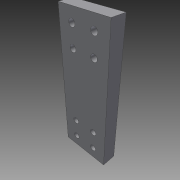
# Autodesk Inventor part: x_iddler_right_cap
Saved by Autodesk Inventor 2014 (Build 180170000, 170)
## iProperties
Created: 2014-03-25
Part Number: x_iddler_right_cap
Material: Plywood, Finish
Document SubType Name: Modeling
Designer: buben
Density: 0.552 g/cm^3
Appearance: Plywood - New
Author: buben
Autodesk Inventor part; units mm, degrees
ref_plane "YZ Plane" through (0, 0, 0) normal (1, 0, 0) x (0, 1, 0)
ref_plane "XZ Plane" through (0, 0, 0) normal (0, 1, 0) x (-1, 0, 0)
ref_plane "XY Plane" through (0, 0, 0) normal (0, 0, 1) x (1, 0, 0)
sketch "Sketch1" plane through (0, 0, 0) normal (0, 1, 0) x (-1, 0, 0)
  line L0 (0, 0) -> (22.5, 0)
  line L1 (22.5, 0) -> (22.5, -62)
  line L2 (22.5, -62) -> (0, -62)
  line L3 (0, -62) -> (0, 0)
  dimension "d0" = 22.5
  dimension "d1" = 62
  constraints: 8 end point, 2 parallel, 1 horizontal, 1 perpendicular
  measures "d0" distance of L0.start L0.end
  measures "d1" distance of L2.end L0.start
extrude "Extrusion1" add sketch "Sketch1" along normal blind 6.5
sketch "Sketch2" plane through (0, 6.5, 0) normal (0, 1, 0) x (1, 0, 0)
  line L0 (0, 62) -> (-22.5, 62) projected
  line L1 (-22.5, 62) -> (-22.5, 0) projected
  circle A0 centre (-16.25, 56.5) radius 1.5
  circle A1 centre (-16.25, 47.5) radius 1.5
  circle A2 centre (-6.25, 56.5) radius 1.5
  circle A3 centre (-6.25, 47.5) radius 1.5
  circle A4 centre (-16.25, 14.5) radius 1.5
  circle A5 centre (-16.25, 5.5) radius 1.5
  circle A6 centre (-6.25, 14.5) radius 1.5
  circle A7 centre (-6.25, 5.5) radius 1.5
  line L2 (-16.25, 56.5) -> (-6.25, 56.5) construction
  line L3 (-16.25, 56.5) -> (-6.25, 47.5) construction
  line L4 (-16.25, 47.5) -> (-6.25, 56.5) construction
  line L5 (-16.25, 14.5) -> (-6.25, 5.5) construction
  line L6 (-6.25, 14.5) -> (-16.25, 5.5) construction
  line L7 (-11.25, 52) -> (-11.25, 10) construction
  point P0 (-11.25, 56.5)
  point P1 (-11.25, 62)
  point P2 (-11.25, 31)
  point P3 (-22.5, 31)
  dimension "d5" = 3
  dimension "d6" = 9
  dimension "d7" = 10
  dimension "d8" = 9
  dimension "d9" = 42
  constraints: 12 end point, 8 centre point, 8 midpoint, 7 equal radius, 7 vertical alignment, 5 horizontal alignment, 1 perpendicular
  measures "d5" diameter of A0
  measures "d6" distance of L4.start L2.start
  measures "d7" distance of L2.start L2.end
  measures "d8" distance of L6.end L5.start
  measures "d9" distance of L7.start point (-11.25, 10)
extrude "Extrusion2" cut sketch "Sketch2" against normal through all
equation "\"d8\" = d6"
body "Solid1"
